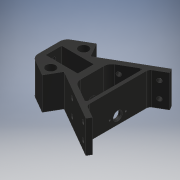
# Autodesk Inventor part: Coins superieur
Saved by Autodesk Inventor 2017 (Build 210142000, 142)
## iProperties
Company: FABLAB Frenchmakers
Part Number: Coins superieur
Material: Aluminium
Document SubType Name: Modeling
Designer: FABLAB Frenchmakers
Density: 2.7 g/cm^3
Appearance: Aluminium - Plat(1)
Mass: 273.076 g
Surface Area: 368.992 cm^2
Volume: 101.139 cm^3
Stock Number: 1420-01-04
Project: 1420 Vauban 3D XL
Catalog Web Link: http://frenchmakers.com/
Autodesk Inventor part; units mm, degrees
note: some values were not read from the file. Chosen so that the rebuilt part matches the saved one: direction of "Maintient profilé vertical".
ref_plane "YZ Plane" through (0, 0, 0) normal (1, 0, 0) x (0, 1, 0)
ref_plane "XZ Plane" through (0, 0, 0) normal (0, 1, 0) x (-1, 0, 0)
ref_plane "XY Plane" through (0, 0, 0) normal (0, 0, 1) x (1, 0, 0)
sketch "Esquisse1" plane through (0, 0, 0) normal (0, 0, 1) x (1, 0, 0)
  line L0 (0, 0) -> (0, 38.6276)
  line L1 (0, 38.6276) -> (16.5, 48.1538)
  line L2 (16.5, 48.1538) -> (13.5, 53.35)
  line L3 (13.5, 53.35) -> (-50.3694, 16.475)
  line L4 (-50.3694, 16.475) -> (-60.3694, 33.7955)
  line L5 (-60.3694, 33.7955) -> (-80.7, 22.0576)
  line L6 (-85.7, 13.3974) -> (-85.7, 0)
  line L7 (-85.7, 0) -> (0, 0)
  arc A0 (-80.7, 22.0576) -> (-85.7, 13.3974) centre (-75.7, 13.3974) ccw
  line L8 (-79.9, 0) -> (-39.75, 0) construction
  line L9 (-39.75, 0) -> (-39.75, 10.075) construction
  line L10 (-39.75, 10.075) -> (-79.9, 10.075) construction
  line L11 (-79.9, 10.075) -> (-79.9, 0) construction
  dimension "d0" = 20
  dimension "d1" = 73.75
  dimension "d3" = 6
  dimension "d4" = 16.5
  dimension "d7" = 85.7
  dimension "d32" = 40.15
  dimension "d33" = 5.8
  dimension "d34" = 10.075
  dimension "d35" = 6.4
  dimension "d38" = 120
  dimension "d39" = 10
  constraints: 24 end point, 5 perpendicular, 4 parallel, 2 point on circle, 2 tangent, 1 centre point, 1 coincident, 1 horizontal, 1 point on line, 1 vertical
  measures "d0" distance of L3.end L4.end
  measures "d1" distance of L2.end L3.end
  measures "d3" distance of L1.end L2.end
  measures "d4" distance from line of L1.end L0
  measures "d7" distance between parallel lines of L0 L6
  measures "d32" distance of L9.end L10.end
  measures "d33" distance between parallel lines of L6 L11
  measures "d34" distance between parallel lines of L8 L10
  measures "d35" distance from line of L3.end L10
  measures "d38" angle of L5 L6
  measures "d39" radius of A0
extrude "Embase" add sketch "Esquisse1" along normal mid plane 40.2
mirror "Symétrie1" about plane through (-85.7, 0, 0) normal (0, -1, 0) of "Embase"
sketch "Esquisse2" plane through (0, 0, 20.1) normal (0, 0, 1) x (1, 0, 0)
  line L0 (-79.95, -10.075) -> (-39.8, -10.075)
  line L1 (-39.8, -10.075) -> (-39.8, 10.075)
  line L2 (-39.8, 10.075) -> (-79.95, 10.075)
  line L3 (-79.95, 10.075) -> (-79.95, -10.075)
  line L4 (0, 38.6276) -> (0, -38.6276) projected
  line L5 (-85.7, 13.3974) -> (-85.7, -13.3974) projected
  point P0 (0, 0)
  point P1 (-39.8, 0)
  point P2 (0, 0)
  dimension "d14" = 20.15
  dimension "d15" = 40.15
  dimension "d16" = 5.75
  constraints: 8 end point, 2 midpoint, 2 parallel, 1 horizontal, 1 horizontal alignment, 1 perpendicular
  measures "d14" distance of L0.end L1.end
  measures "d15" distance of L1.end L2.end
  measures "d16" distance between parallel lines of L5 L3
extrude "Passage profilé vertical" cut sketch "Esquisse2" against normal through all
sketch "Esquisse3" plane through (0, 0, 20.1) normal (0, 0, 1) x (1, 0, 0)
  line L0 (-31.8, -20.3371) -> (-31.8, 20.3371)
  line L1 (-31.8, 20.3371) -> (-3.9, 36.4452)
  line L2 (-3.9, 36.4452) -> (-3.9, -36.4452)
  line L3 (-31.8, -20.3371) -> (-3.9, -36.4452)
  line L4 (0, 38.6276) -> (0, -38.6276) projected
  line L5 (13.5, 53.35) -> (-50.3694, 16.475) projected
  line L6 (13.5, -53.35) -> (-50.3694, -16.475) projected
  point P0 (0, 0)
  dimension "d19" = 27.9
  dimension "d20" = 3.9
  dimension "d21" = 5.94
  dimension "d22" = 5.94
  constraints: 8 end point, 2 parallel, 1 equal length, 1 vertical
  measures "d19" distance between parallel lines of L2 L0
  measures "d20" distance between parallel lines of L4 L2
  measures "d21" distance between parallel lines of L5 L1
  measures "d22" distance between parallel lines of L6 L3
extrude "Passage courroie" cut sketch "Esquisse3" against normal through all
fillet "Congé1" radius 10 2 edges at (-31.8, -20.3371, 0) (-31.8, 20.3371, 0)
fillet "Congé1" radius 2 2 edges at (-3.9, -36.4452, 0) (-3.9, 36.4452, 0)
fillet "Congé1" radius 5 2 edges at (0, -38.6276, 0) (0, 38.6276, 0)
sketch "Esquisse7" plane through (0, 0, 20.1) normal (0, 0, 1) x (1, 0, 0)
  point P0 (0, 0)
  point P1 (-63, -20.5)
  point P2 (-63, 20.5)
  dimension "d51" = 20.5
  dimension "d52" = 63
  dimension "d53" = 20.5
  dimension "d54" = 63
  measures "d51" vertical distance of point (0, 0) point (-63, -20.5)
  measures "d52" horizontal distance of point (0, 0) point (-63, -20.5)
  measures "d53" vertical distance of point (0, 0) point (-63, 20.5)
  measures "d54" horizontal distance of point (0, 0) point (-63, 20.5)
hole "Passage axe" at (-63, -20.5, 20.1) at (-63, 20.5, 20.1) direction (0, 0, -1) diameter 12 end through all
sketch "Esquisse8" plane through (-85.7, 13.3974, -20.1) normal (-1, 0, 0) x (0, 0, 1)
  point P0 (20.1, -13.3974)
  point P1 (10.1, -13.3974)
  point P2 (30.1, -13.3974)
  dimension "d55" = 20
  dimension "d56" = 10
  constraints: 2 horizontal alignment
  measures "d55" distance of point (10.1, -13.397) point (30.1, -13.397)
  measures "d56" distance of point (20.1, -13.397) point (30.1, -13.397)
hole "Maintient profilé vertical" at (-85.7, 0, -10) at (-85.7, 0, 10) direction (1, 0, 0) diameter 5.5 end up to surface countersink diameter 9.5 countersink angle 90
sketch "Esquisse9" plane through (-50.3694, -16.475, -20.1) normal (-0.5, -0.8660254, 0) x (0.8660254, -0.5, 0)
  line L0 (0, 0) -> (73.75, 0) projected
  line L1 (73.75, 40.2) -> (0, 40.2) projected
  line L2 (73.75, 40.2) -> (73.75, 0) projected
  point P0 (35.3837, 20.1)
  point P1 (27.3, 30.1)
  point P2 (27.3, 10.3)
  point P3 (64.5, 30.1)
  point P4 (64.5, 10.3)
  dimension "d64" = 37.2
  dimension "d66" = 10.3
  dimension "d67" = 10.1
  dimension "d68" = 9.25
  constraints: 2 horizontal alignment, 2 vertical alignment
  measures "d64" distance of point (64.5, 10.3) point (27.3, 10.3)
  measures "d66" distance from line of L0 point (64.5, 10.3)
  measures "d67" distance from line of L1 point (64.5, 30.1)
  measures "d68" distance from line of L2 point (64.5, 30.1)
hole "Maintient profilé horizonal" at (-26.7269, -30.125, 10) at (-26.7269, -30.125, -9.8) at (5.4893, -48.725, 10) at (5.4893, -48.725, -9.8) direction (0.5, 0.8660254, 0) diameter 5.2 depth 8 tip angle 118
mirror "Symétrie2" about plane through (0, 0, 0) normal (0, 1, 0) of "Maintient profilé horizonal"
sketch "Esquisse10" plane through (0, -35.7408, 20.1) normal (1, 0, 0) x (0, 0, -1)
  line L0 (40.2, 71.4816) -> (40.2, 0) projected
  point P0 (20.1, 35.7408)
  point P1 (30.6, 35.7408)
  dimension "d76" = 9.6
  constraints: 1 horizontal alignment
  measures "d76" distance from line of L0 point (30.6, 35.741)
hole "Perçage roulement a bille" at (0, 0, -10.5) direction (-1, 0, 0) diameter 10 depth 10 tip angle 118 counterbore diameter 11.5 counterbore depth 1
sketch "Esquisse11" plane through (0, -35.7408, 20.1) normal (1, 0, 0) x (0, 0, -1)
  circle A0 centre (30.6, 35.7408) radius 5 construction
  point P0 (20.1, 35.7408)
  point P1 (30.6, 25.7408)
  point P2 (30.6, 45.7408)
  dimension "d84" = 20
  dimension "d85" = 10
  constraints: 2 vertical alignment
  measures "d84" distance of point (30.6, 25.741) point (30.6, 45.741)
  measures "d85" distance of A0.centre point (30.6, 25.741)
hole "Taraudage plaque de maintient" at (0, -10, -10.5) at (0, 10, -10.5) direction (-1, 0, 0) diameter 2.013 depth 7.6 tip angle 118 thread size "M2.5x0.45" class "6H" standard "ISO Metric profile"
sketch "Esquisse12" plane through (-31.8, -14.5636, 20.1) normal (1, 0, 0) x (0, 0, -1)
  circle A0 centre (30.6, 14.5636) radius 5 construction
  point P0 (20.1, 14.5636)
  constraints: 1 coincident
hole "Perçage roulement a bille intérieur" at (-31.8, 0, -10.5) direction (-1, 0, 0) diameter 10.5 depth 3
equation "\"d22\" = d21"
equation "\"d53\" = d51"
equation "\"d54\" = d52"
equation "\"d56\" = 0.5 * d55"
equation "\"d85\" = 0.5 * d84"
